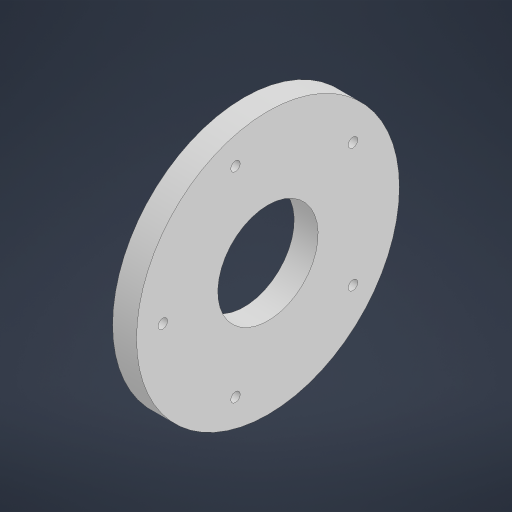
# Autodesk Inventor part: panel bushing support
Saved by Autodesk Inventor 2023.2 (Build 272271030, 271C)
## iProperties
Created: 2023-04-05
Part Number: panel bushing support
Material: Generic
Document SubType Name: Modeling
Designer: ralph
Density: 1 g/cm^3
Appearance: Default
Author: ralph
Autodesk Inventor part; units mm, degrees
ref_plane "YZ Plane" through (0, 0, 0) normal (1, 0, 0) x (0, 1, 0)
ref_plane "XZ Plane" through (0, 0, 0) normal (0, 1, 0) x (-1, 0, 0)
ref_plane "XY Plane" through (0, 0, 0) normal (0, 0, 1) x (1, 0, 0)
sketch "Sketch1" plane through (0, 0, 0) normal (1, 0, 0) x (0, 1, 0)
  circle A0 centre (0, 0) radius 13.335
  circle A1 centre (0, 0) radius 34.925
  circle A2 centre (0, 27.94) radius 1.27
  circle A3 centre (0, 0) radius 27.94
  circle A4 centre (26.5725, 8.6339) radius 1.27
  circle A5 centre (16.4227, -22.6039) radius 1.27
  circle A6 centre (-16.4227, -22.6039) radius 1.27
  circle A7 centre (-26.5725, 8.6339) radius 1.27
  dimension "d4" = 55.88
  dimension "d0" = 26.67
  dimension "d1" = 69.85
  dimension "d2" = 2.54
  dimension "d7" = 360
  constraints: 7 centre point, 5 coincident, 1 vertical alignment, 16 other
  measures "d0" diameter of A0
  measures "d1" diameter of A1
  measures "d2" diameter of A2
extrude "Extrusion1" add sketch "Sketch1" along normal blind 6.35 contours A1 | A2 A3 A4 A5 A6 A7
body "Solid1"
